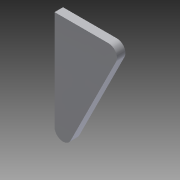
# Autodesk Inventor part: Gusset Connector 2
Saved by Autodesk Inventor 2013 (Build 170138000, 138)
## iProperties
Created: 2013-01-26
Part Number: Gusset Connector 2
Material: Aluminum 6061
Document SubType Name: Modeling
Designer: actoennies
Mass: 5.24772 g
Surface Area: 15.7154 cm^2
Volume: 1.93643 cm^3
Density: 2.71 g/cm^3
Author: actoennies
Autodesk Inventor part; units mm, degrees
ref_plane "YZ Plane" through (0, 0, 0) normal (1, 0, 0) x (0, 1, 0)
ref_plane "XZ Plane" through (0, 0, 0) normal (0, 1, 0) x (-1, 0, 0)
ref_plane "XY Plane" through (0, 0, 0) normal (0, 0, 1) x (1, 0, 0)
sketch "Sketch1" plane through (0, 0, 0) normal (0, 0, 1) x (1, 0, 0)
  line L0 (0, 13.4495) -> (0, 50.8)
  line L1 (0, 50.8) -> (20.2627, 50.8)
  line L2 (23.1025, 46.2051) -> (6.0148, 12.0296)
  arc A0 (0, 13.4495) -> (6.0148, 12.0296) centre (3.175, 13.4495) ccw
  arc A1 (23.1025, 46.2051) -> (20.2627, 50.8) centre (20.2627, 47.625) ccw
  point P0 (0, 0)
  point P1 (25.4, 50.8)
  dimension "d0" = 50.8
  dimension "d1" = 25.4
  dimension "d2" = 3.175
  dimension "d3" = 3.175
  constraints: 6 end point, 4 point on circle, 4 point on line, 4 tangent, 2 centre point, 1 perpendicular, 1 vertical
  measures "d0" distance of point (0, 0) L0.end
  measures "d1" distance of L0.end point (25.4, 50.8)
  measures "d2" radius of A0
  measures "d3" radius of A1
extrude "Extrusion1" add sketch "Sketch1" along normal blind 3.175
body "Solid1"
